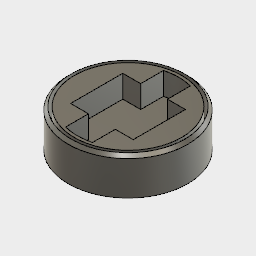
ANS0016_static_bottom v3 (Autodesk Fusion 360 design; units mm, degrees)
Autodesk Fusion 360 part; units mm, degrees
sketch "Sketch1" plane through (0, 0, 0) normal (0, 1, 0) x (1, 0, 0)
  circle A0 centre (0, 0) radius 40
  dimension "d1" = 80
  measures "d1" diameter of A0
extrude "Extrude1" add sketch "Sketch1" along normal blind 25
sketch "Sketch2" plane through (0, 25, 0) normal (0, 1, 0) x (-1, 0, 0)
  circle A0 centre (0, 0) radius 40
  circle A1 centre (0, 0) radius 38
  circle A2 centre (0, 0) radius 36
  dimension "d4" = 76
  dimension "d5" = 72
  measures "d4" diameter of A1
  measures "d5" diameter of A2
extrude "Extrude2" cut sketch "Sketch2" against normal blind 15 contours A1
sketch "Sketch3" plane through (0, 25, 0) normal (0, 1, 0) x (-1, 0, 0)
  circle A0 centre (0, 0) radius 36
  circle A1 centre (0, 0) radius 34
  circle A2 centre (0, 0) radius 32
  line L0 (21, 17.5) -> (-21, 17.5)
  line L1 (-21, 17.5) -> (-21, -17.5)
  line L2 (-21, -17.5) -> (21, -17.5)
  line L3 (21, -17.5) -> (21, 17.5)
  line L4 (21, 17.5) -> (-21, -17.5) construction
  line L5 (-21, 17.5) -> (21, -17.5) construction
  line L6 (0, 0) -> (9, 0)
  line L7 (0, 0) -> (-9, 0)
  line L8 (9, 0) -> (9, -32.7872)
  line L9 (-9, 0) -> (-9, -32.7872)
  line L10 (9, 0) -> (9, 32.7872)
  line L11 (-9, 0) -> (-9, 32.7872)
  dimension "d8" = 68
  dimension "d9" = 64
  dimension "d10" = 42
  dimension "d11" = 35
  dimension "d12" = 9
  dimension "d13" = 9
  constraint perpendicular L0 L1
  constraint parallel L0 L2
  constraint parallel L1 L3
  constraint horizontal L0
  constraint coincident L4
  constraint coincident L5
  constraint coincident A1
  constraint perpendicular L2 L8
  constraint perpendicular L7 L9
  constraint perpendicular L0 L10
  constraint perpendicular L0 L11
  measures "d8" diameter of A1
  measures "d9" diameter of A2
extrude "Extrude3" cut sketch "Sketch3" against normal blind 15 contours A1 A2 L10 L11 | A1 A2 L8 L9 | A2 L0 L10 L11 | A2 L2 L8 L9 | L0 L6 L7 L10 L11 | L0 L2 L3 L8 L10 | L2 L6 L7 L8 L9 | L0 L1 L2 L9 L11
chamfer "Chamfer1" distance 2 angle 45 1 edges at (-37.2931, 25, 14.4646)
